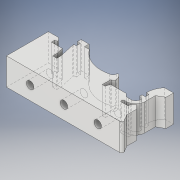
# Autodesk Inventor part: DINRailAdapter_PhoenixContact_1201578
Saved by Autodesk Inventor 2019.1 (Build 231200000, 200)
## iProperties
Created: 2018-10-29
Part Number: DINRailAdapter_PhoenixContact_1201578
Material: PC/ABS Plastic
Document SubType Name: Modeling
Designer: huesof
Density: 0.357273 g/cm^3
Appearance: Smooth - White
Mass: 1.98001 g
Surface Area: 28.826 cm^2
Volume: 5.54201 cm^3
Author: huesof
Autodesk Inventor part; units mm, degrees
ref_plane "YZ Plane" through (0, 0, 0) normal (1, 0, 0) x (0, 1, 0)
ref_plane "XZ Plane" through (0, 0, 0) normal (0, 1, 0) x (-1, 0, 0)
ref_plane "XY Plane" through (0, 0, 0) normal (0, 0, 1) x (1, 0, 0)
sketch "Sketch1" plane through (0, 0, 0) normal (0, 1, 0) x (-1, 0, 0)
  line L0 (0, 0) -> (21.245, 0)
  line L1 (0, 0) -> (-20.6799, 0)
  line L2 (-21.2644, -1.0125) -> (-19.895, -3.3844)
  line L3 (-21.849, 0) -> (-19.1101, 0) construction
  arc A0 (-20.6799, 0) -> (-21.2644, -1.0125) centre (-20.6799, -0.675) ccw
  line L4 (-19.895, -3.3844) -> (-19.895, -6.9494)
  line L5 (-19.895, -6.9494) -> (-18.415, -8.4294)
  line L6 (-19.895, -6.9494) -> (-17.802, -6.9494) construction
  line L7 (-18.415, -8.4294) -> (-17.295, -7.3093)
  line L8 (-17.295, -7.3093) -> (-17.295, -6.4493)
  line L9 (-17.295, -6.4493) -> (-14.828, -6.4493)
  line L10 (-14.303, -6.9743) -> (-14.303, -6.9743)
  line L11 (-14.828, -7.4993) -> (-15.608, -7.4993)
  arc A1 (-14.303, -6.9743) -> (-14.828, -6.4493) centre (-14.828, -6.9743) ccw
  arc A2 (-14.828, -7.4993) -> (-14.303, -6.9743) centre (-14.828, -6.9743) ccw
  arc A3 (-15.608, -7.4993) -> (-19.008, -10.8993) centre (-15.608, -10.8993) ccw
  line L12 (-15.608, -10.8993) -> (-19.008, -10.8993) construction
  line L13 (-15.608, -10.8993) -> (-15.608, -7.4993) construction
  line L14 (-19.008, -10.8993) -> (-19.008, -14.7753)
  line L15 (-19.008, -14.7753) -> (-21.5082, -16.2188)
  line L16 (-19.008, -14.7753) -> (-16.121, -14.7753) construction
  line L17 (-21.5082, -16.2188) -> (-21.5082, -19.0078)
  line L18 (-21.5082, -19.0078) -> (-18.2032, -19.0078)
  line L19 (-18.2032, -19.0078) -> (-16.4072, -19.0078) construction
  line L20 (-16.4072, -19.0078) -> (-16.4072, -14.1078) construction
  line L21 (-16.4072, -14.1078) -> (-17.4338, -13.9075)
  line L22 (-16.4072, -14.1078) -> (-15.3612, -14.1078) construction
  line L23 (-17.4338, -13.9075) -> (-17.5463, -12.5572)
  line L24 (-17.4338, -13.9075) -> (-16.0788, -13.9075) construction
  line L25 (-17.5463, -12.5572) -> (-16.2583, -12.5572)
  line L26 (-16.2583, -12.5572) -> (-16.2583, -11.8072)
  line L27 (-16.2583, -11.8072) -> (-17.5081, -11.2244)
  line L28 (-17.5081, -11.2244) -> (-17.5081, -10.7074)
  line L29 (-15.8081, -9.0074) -> (-14.8361, -9.0074)
  arc A4 (-15.8081, -9.0074) -> (-17.5081, -10.7074) centre (-15.8081, -10.7074) ccw
  line L30 (-14.8361, -9.0074) -> (-12.9081, -9.0074) construction
  line L31 (-12.9081, -9.0074) -> (-12.9081, -10.1074) construction
  line L32 (-12.9081, -10.1074) -> (-13.4221, -9.5934)
  line L33 (-12.9081, -10.1074) -> (-12.1811, -10.1074) construction
  line L34 (-12.9081, -10.1074) -> (-7.1081, -10.1074)
  line L35 (-7.1081, -10.1074) -> (-6.6795, -8.5079)
  line L36 (-7.1081, -10.1074) -> (-5.4521, -10.1074) construction
  line L37 (-6.6795, -8.5079) -> (-5.6835, -8.5079)
  line L38 (-5.6835, -8.5079) -> (-5.6835, -11.7279)
  line L39 (-5.6835, -11.7279) -> (-5.9885, -11.7279) construction
  line L40 (-5.9885, -11.7279) -> (-5.9885, -12.3579) construction
  arc A5 (-5.6835, -11.7279) -> (-6.6884, -12.3579) centre (-5.9885, -12.3579) ccw
  line L41 (-5.6835, -11.7279) -> (-5.2885, -11.7279) construction
  line L42 (-5.2885, -11.7279) -> (-5.2885, -14.4619) construction
  line L43 (-5.6835, -11.7279) -> (-3.3405, -11.7279) construction
  line L44 (-3.3405, -11.7279) -> (-3.3405, -12.2459) construction
  line L45 (-5.6835, -11.7279) -> (-5.5525, -11.7279) construction
  line L46 (-5.5525, -11.7279) -> (-5.5525, -14.7619) construction
  arc A6 (-5.5525, -14.7624) -> (-4.8885, -14.4619) centre (-5.2885, -14.4619) ccw
  line L47 (-5.6835, -11.7279) -> (7.9675, -11.7279) construction
  line L48 (7.9675, -11.7279) -> (7.9675, -17.3579) construction
  arc A7 (-3.6885, -13.2619) -> (-4.8885, -14.4619) centre (-3.6885, -14.4619) ccw
  line L49 (-3.6885, -14.4619) -> (-3.6885, -13.2619) construction
  line L50 (-3.6885, -14.4619) -> (-4.8885, -14.4619) construction
  arc A8 (7.9675, -17.3579) -> (-3.6885, -13.2619) centre (-0.878, -23.8967) ccw
  line L51 (7.9675, -17.3579) -> (9.7415, -17.3579)
  line L52 (9.7415, -17.3579) -> (9.7415, -19.0079)
  line L53 (9.7415, -19.0079) -> (12.6915, -19.0079)
  line L54 (12.6915, -19.0079) -> (12.6915, -17.7329)
  line L55 (12.6915, -17.7329) -> (11.5413, -17.6079)
  line L56 (11.5413, -17.6079) -> (11.5413, -16.1079)
  line L57 (11.5413, -16.1079) -> (12.3913, -16.1079)
  line L58 (12.3913, -16.1079) -> (12.3913, -15.6079)
  line L59 (12.3913, -15.6079) -> (11.1663, -10.0821)
  line L60 (11.1663, -10.0821) -> (11.1663, -8.5081)
  line L61 (11.1663, -8.5081) -> (12.6663, -8.5081)
  line L62 (12.6663, -8.5081) -> (12.6915, -10.3399)
  line L63 (12.6915, -10.3399) -> (13.2493, -12.7009)
  line L64 (13.2493, -12.7009) -> (17.3243, -12.7009)
  line L65 (17.3243, -12.7009) -> (17.3243, -13.9009)
  line L66 (17.3243, -13.9009) -> (16.5239, -14.1011)
  line L67 (16.5239, -14.1011) -> (16.5239, -14.5511)
  line L68 (16.5239, -14.5511) -> (17.4743, -15.5014)
  line L69 (17.4743, -15.5014) -> (21.245, -15.5014)
  line L70 (21.245, -15.5014) -> (21.245, 0)
  arc A9 (-18.2032, -19.0078) -> (-16.4072, -14.1078) centre (-23.8069, -14.1748) ccw
  arc A10 (-13.4221, -9.5934) -> (-14.8361, -9.0074) centre (-14.8365, -11.0074) ccw
  arc A11 (-6.6884, -12.3579) -> (-5.5525, -14.7624) centre (-3.3403, -12.2467) ccw
  point P0 (-14.303, -6.4493)
  point P1 (-14.303, -7.4993)
  point P2 (-17.5081, -9.0074)
  dimension "d0" = 21.245
  dimension "d1" = 21.849
  dimension "d2" = 3.908
  dimension "d3" = 60
  dimension "d4" = 0.675
  dimension "d5" = 3.565
  dimension "d6" = 45
  dimension "d7" = 2.093
  dimension "d8" = 1.584
  dimension "d9" = 0.86
  dimension "d10" = 2.992
  dimension "d11" = 1.05
  dimension "d12" = 1.305
  dimension "d13" = 0.525
  dimension "d14" = 90
  dimension "d15" = 3.4
  dimension "d16" = 3.876
  dimension "d17" = 2.887
  dimension "d18" = 150
  dimension "d19" = 2.789
  dimension "d20" = 3.305
  dimension "d21" = 1.796
  dimension "d22" = 4.9
  dimension "d25" = 1.046
  dimension "d26" = 168.96
  dimension "d27" = 265.24
  dimension "d28" = 1.355
  dimension "d29" = 1.288
  dimension "d30" = 0.75
  dimension "d31" = 1.379
  dimension "d32" = 115
  dimension "d33" = 2.217
  dimension "d35" = 2.672
  dimension "d36" = 1.7
  dimension "d37" = 1.928
  dimension "d38" = 1.1
  dimension "d39" = 0.727
  dimension "d40" = 135
  dimension "d41" = 5.8
  dimension "d44" = 1.656
  dimension "d45" = 75
  dimension "d46" = 0.996
  dimension "d47" = 3.22
  dimension "d48" = 0.305
  dimension "d49" = 0.63
  dimension "d50" = 0.395
  dimension "d51" = 2.734
  dimension "d52" = 2.343
  dimension "d53" = 0.518
  dimension "d54" = 0.131
  dimension "d55" = 3.034
  dimension "d57" = 0.4
  dimension "d58" = 13.651
  dimension "d59" = 5.63
  dimension "d60" = 90
  dimension "d61" = 1.2
  dimension "d62" = 0
  dimension "d63" = 11
  dimension "d64" = 1.774
  dimension "d65" = 1.65
  dimension "d66" = 2.95
  dimension "d67" = 1.275
  dimension "d68" = 1.157
  dimension "d69" = 96.2
  constraints: 142 end point, 25 perpendicular, 24 point on circle, 17 horizontal, 14 point on line, 12 centre point, 8 tangent, 7 equal length, 5 parallel, 4 vertical, 2 coincident, 1 concentric
  measures "d0" distance of L0.start L0.end
  measures "d1" distance of L0.start L3.start
  measures "d2" distance of L3.start L2.end
  measures "d3" angle of L2 L3
  measures "d4" radius of A0
  measures "d5" distance of L2.end L4.end
  measures "d6" angle of L5 L6
  measures "d7" distance of L4.end L5.end
  measures "d8" distance of L5.end L7.end
  measures "d9" distance of L7.end L8.end
  measures "d10" distance of L8.end point (-14.303, -6.449)
  measures "d11" distance of point (-14.303, -6.449) point (-14.303, -7.499)
  measures "d12" distance of point (-14.303, -7.499) L11.end
  measures "d13" radius of A1
  measures "d14" angle of L13 L12
  measures "d15" distance of L12.start L11.end
  measures "d16" distance of L12.end L14.end
  measures "d17" distance of L14.end L15.end
  measures "d18" angle of L15 L16
  measures "d19" distance of L15.end L17.end
  measures "d20" distance of L17.end L18.end
  measures "d21" distance of L18.end L19.end
  measures "d22" distance of L19.end L20.end
  measures "d25" distance of L20.end L21.end
  measures "d26" angle of L22 L21
  measures "d28" distance of L21.end L23.end
  measures "d29" distance of L23.end L25.end
  measures "d30" distance of L25.end L26.end
  measures "d31" distance of L26.end L27.end
  measures "d32" angle of L27 L26
  measures "d33" distance of L27.end point (-17.508, -9.007)
  measures "d35" distance of point (-17.508, -9.007) L29.end
  measures "d36" radius of A4
  measures "d37" distance of L29.end L30.end
  measures "d38" distance of L30.end L31.end
  measures "d39" distance of L31.end L32.end
  measures "d40" angle of L33 L32
  measures "d41" distance of L31.end L34.end
  measures "d44" distance of L34.end L35.end
  measures "d45" angle of L36 L35
  measures "d46" distance of L35.end L37.end
  measures "d47" distance of L37.end L38.end
  measures "d48" distance of L38.end L39.end
  measures "d49" distance of L39.end L40.end
  measures "d50" distance of L38.end L41.end
  measures "d51" distance of L41.end L42.end
  measures "d52" distance of L38.end L43.end
  measures "d53" distance of L43.end L44.end
  measures "d54" distance of L38.end L45.end
  measures "d55" distance of L45.end L46.end
  measures "d57" radius of A6
  measures "d58" distance of L38.end L47.end
  measures "d59" distance of L47.end L48.end
  measures "d60" angle of L49 L50
  measures "d61" distance of L50.end L49.start
  measures "d62" vertical distance of L42.end L50.end
  measures "d63" radius of A8
  measures "d64" distance of L48.end L51.end
  measures "d65" distance of L51.end L52.end
  measures "d66" distance of L52.end L53.end
  measures "d67" distance of L53.end L54.end
  measures "d68" distance of L54.end L55.end
  measures "d69" angle of L55 L54
extrude "Extrusion1" add sketch "Sketch1" along normal blind 5 and the other way blind 5
sketch "Sketch2" plane through (0, 0, 0) normal (0, 0, 1) x (1, 0, 0)
  point P0 (0, 0)
  point P1 (0, 0)
  point P2 (12.5, 0)
  point P3 (-12.5, 0)
  dimension "d95" = 12.5
  dimension "d96" = 12.5
  dimension "d97" = 0
  dimension "d98" = 0
  constraints: 1 coincident
  measures "d95" distance of point (0, 0) point (-12.5, 0)
  measures "d96" distance of point (12.5, 0) point (0, 0)
  measures "d97" vertical distance of point (0, 0) point (12.5, 0)
  measures "d98" vertical distance of point (-12.5, 0) point (0, 0)
hole "Hole1" at (0, 0, 0) at (12.5, 0, 0) at (-12.5, 0, 0) direction (0, 0, -1) diameter 2.75 depth 7.35
body "Solid1"
